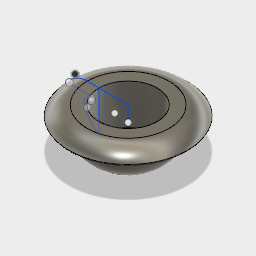
Joint_dia_16mm v1 (Autodesk Fusion 360 design; units mm, degrees)
Autodesk Fusion 360 part; units mm, degrees
sketch "Sketch2" plane through (0, 0, 0) normal (0, 0, 1) x (1, 0, 0)
  line L0 (43.6, 58) -> (42, 58)
  line L1 (42, 58) -> (40.3449, 58)
  line L2 (35.1446, 55.2169) -> (35.2591, 55.3887)
  line L3 (35.4671, 55) -> (41.5, 55)
  line L4 (42, 54.5) -> (42, 53.9)
  line L5 (41.5, 53.4) -> (39.5, 53.4)
  line L6 (43.5926, 46.8889) -> (43.6, 58)
  arc A0 (39.5, 53.4) -> (43.5926, 46.8889) centre (47.9075, 54.1428) ccw
  arc A1 (42, 54.5) -> (41.5, 55) centre (41.5, 54.5) ccw
  arc A2 (41.5, 53.4) -> (42, 53.9) centre (41.5, 53.9) ccw
  arc A3 (40.3449, 58) -> (35.1446, 55.2169) centre (40.3449, 51.75) ccw
  arc A4 (35.2591, 55.3887) -> (35.4671, 55) centre (35.4671, 55.25) ccw
  line L7 (43.6, 58) -> (51.6, 57.9946)
  line L8 (51.6, 57.9946) -> (51.5972, 53.7744)
  point P0 (37, 58)
  dimension "d9" = 1.6
  dimension "d10" = 5
  dimension "d12" = 3
  dimension "d13" = 1.6
  dimension "d15" = 5
  dimension "d18" = 0.5
  dimension "d19" = 0.5
  dimension "d20" = 6.25
  dimension "d21" = 0.25
  dimension "d22" = 8
  measures "d9" distance of L0.start L0.end
  measures "d10" distance of L0.end P0
  measures "d12" distance of L1 L3
  measures "d13" distance of L3 L5
  measures "d15" distance of P0 L4
  measures "d18" radius of A1
  measures "d19" radius of A2
  measures "d20" radius of A3
  measures "d21" radius of A4
  measures "d22" distance of L0.start L7.end
revolve "Revolve1" add sketch "Sketch2" angle 360 about axis through (51.6, 57.9946, 0) along (-0.00067, -1, 0) contours L0 L1 L3 L4 L5 L6 A0 A1 A2 A3 A4
